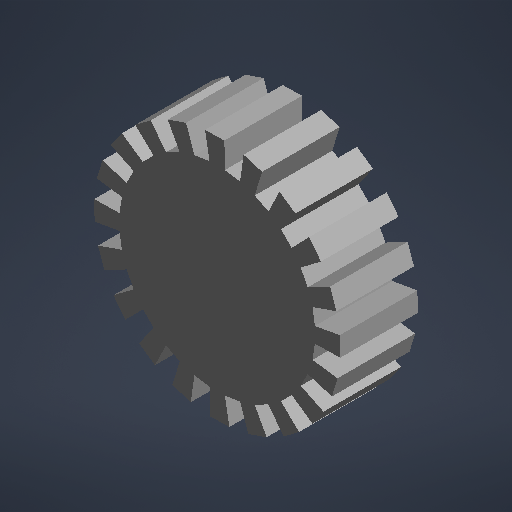
# Autodesk Inventor part: pinn_optimized_geometry
Saved by Autodesk Inventor 2027 (Build 310192060, 192F)
## iProperties
Part Number: pinn_optimized_geometry
Material: Generic
Document SubType Name: Modeling
Designer: altug
Appearance: Default
Author: altug
Required_Hardness: 398.64344334602356
Autodesk Inventor part; units mm, degrees
ref_plane "YZ Plane" through (0, 0, 0) normal (1, 0, 0) x (0, 1, 0)
ref_plane "XZ Plane" through (0, 0, 0) normal (0, 1, 0) x (-1, 0, 0)
ref_plane "XY Plane" through (0, 0, 0) normal (0, 0, 1) x (1, 0, 0)
sketch "Gear_Profile_Sketch" plane through (0, 0, 0) normal (0, 0, 1) x (1, 0, 0)
  line L0 (17.4461, -1.373) -> (21.9623, -1.2871)
  line L1 (21.9623, -1.2871) -> (21.8933, 2.1644)
  line L2 (21.8933, 2.1644) -> (17.4461, 1.373)
  line L3 (17.4461, 1.373) -> (17.0165, 4.0853)
  line L4 (17.0165, 4.0853) -> (21.2852, 5.5626)
  line L5 (21.2852, 5.5626) -> (20.1529, 8.8238)
  line L6 (20.1529, 8.8238) -> (16.1679, 6.697)
  line L7 (16.1679, 6.697) -> (14.9212, 9.1437)
  line L8 (14.9212, 9.1437) -> (18.5244, 11.8678)
  line L9 (18.5244, 11.8678) -> (16.4398, 14.6196)
  line L10 (16.4398, 14.6196) -> (13.3071, 11.3653)
  line L11 (13.3071, 11.3653) -> (11.3653, 13.3071)
  line L12 (11.3653, 13.3071) -> (13.9504, 17.0113)
  line L13 (13.9504, 17.0113) -> (11.1175, 18.9842)
  line L14 (11.1175, 18.9842) -> (9.1437, 14.9212)
  line L15 (9.1437, 14.9212) -> (6.697, 16.1679)
  line L16 (6.697, 16.1679) -> (8.0109, 20.4897)
  line L17 (8.0109, 20.4897) -> (4.707, 21.4906)
  line L18 (4.707, 21.4906) -> (4.0853, 17.0165)
  line L19 (4.0853, 17.0165) -> (1.373, 17.4461)
  line L20 (1.373, 17.4461) -> (1.2871, 21.9623)
  line L21 (1.2871, 21.9623) -> (-2.1644, 21.8933)
  line L22 (-2.1644, 21.8933) -> (-1.373, 17.4461)
  line L23 (-1.373, 17.4461) -> (-4.0853, 17.0165)
  line L24 (-4.0853, 17.0165) -> (-5.5626, 21.2852)
  line L25 (-5.5626, 21.2852) -> (-8.8238, 20.1529)
  line L26 (-8.8238, 20.1529) -> (-6.697, 16.1679)
  line L27 (-6.697, 16.1679) -> (-9.1437, 14.9212)
  line L28 (-9.1437, 14.9212) -> (-11.8678, 18.5244)
  line L29 (-11.8678, 18.5244) -> (-14.6196, 16.4398)
  line L30 (-14.6196, 16.4398) -> (-11.3653, 13.3071)
  line L31 (-11.3653, 13.3071) -> (-13.3071, 11.3653)
  line L32 (-13.3071, 11.3653) -> (-17.0113, 13.9504)
  line L33 (-17.0113, 13.9504) -> (-18.9842, 11.1175)
  line L34 (-18.9842, 11.1175) -> (-14.9212, 9.1437)
  line L35 (-14.9212, 9.1437) -> (-16.1679, 6.697)
  line L36 (-16.1679, 6.697) -> (-20.4897, 8.0109)
  line L37 (-20.4897, 8.0109) -> (-21.4906, 4.707)
  line L38 (-21.4906, 4.707) -> (-17.0165, 4.0853)
  line L39 (-17.0165, 4.0853) -> (-17.4461, 1.373)
  line L40 (-17.4461, 1.373) -> (-21.9623, 1.2871)
  line L41 (-21.9623, 1.2871) -> (-21.8933, -2.1644)
  line L42 (-21.8933, -2.1644) -> (-17.4461, -1.373)
  line L43 (-17.4461, -1.373) -> (-17.0165, -4.0853)
  line L44 (-17.0165, -4.0853) -> (-21.2852, -5.5626)
  line L45 (-21.2852, -5.5626) -> (-20.1529, -8.8238)
  line L46 (-20.1529, -8.8238) -> (-16.1679, -6.697)
  line L47 (-16.1679, -6.697) -> (-14.9212, -9.1437)
  line L48 (-14.9212, -9.1437) -> (-18.5244, -11.8678)
  line L49 (-18.5244, -11.8678) -> (-16.4398, -14.6196)
  line L50 (-16.4398, -14.6196) -> (-13.3071, -11.3653)
  line L51 (-13.3071, -11.3653) -> (-11.3653, -13.3071)
  line L52 (-11.3653, -13.3071) -> (-13.9504, -17.0113)
  line L53 (-13.9504, -17.0113) -> (-11.1175, -18.9842)
  line L54 (-11.1175, -18.9842) -> (-9.1437, -14.9212)
  line L55 (-9.1437, -14.9212) -> (-6.697, -16.1679)
  line L56 (-6.697, -16.1679) -> (-8.0109, -20.4897)
  line L57 (-8.0109, -20.4897) -> (-4.707, -21.4906)
  line L58 (-4.707, -21.4906) -> (-4.0853, -17.0165)
  line L59 (-4.0853, -17.0165) -> (-1.373, -17.4461)
  line L60 (-1.373, -17.4461) -> (-1.2871, -21.9623)
  line L61 (-1.2871, -21.9623) -> (2.1644, -21.8933)
  line L62 (2.1644, -21.8933) -> (1.373, -17.4461)
  line L63 (1.373, -17.4461) -> (4.0853, -17.0165)
  line L64 (4.0853, -17.0165) -> (5.5626, -21.2852)
  line L65 (5.5626, -21.2852) -> (8.8238, -20.1529)
  line L66 (8.8238, -20.1529) -> (6.697, -16.1679)
  line L67 (6.697, -16.1679) -> (9.1437, -14.9212)
  line L68 (9.1437, -14.9212) -> (11.8678, -18.5244)
  line L69 (11.8678, -18.5244) -> (14.6196, -16.4398)
  line L70 (14.6196, -16.4398) -> (11.3653, -13.3071)
  line L71 (11.3653, -13.3071) -> (13.3071, -11.3653)
  line L72 (13.3071, -11.3653) -> (17.0113, -13.9504)
  line L73 (17.0113, -13.9504) -> (18.9842, -11.1175)
  line L74 (18.9842, -11.1175) -> (14.9212, -9.1437)
  line L75 (14.9212, -9.1437) -> (16.1679, -6.697)
  line L76 (16.1679, -6.697) -> (20.4897, -8.0109)
  line L77 (20.4897, -8.0109) -> (21.4906, -4.707)
  line L78 (21.4906, -4.707) -> (17.0165, -4.0853)
  line L79 (17.0165, -4.0853) -> (17.4461, -1.373)
  constraints: 160 end point
extrude "Extrusion1" add sketch "Gear_Profile_Sketch" against normal blind 13.86
body "Solid1"
